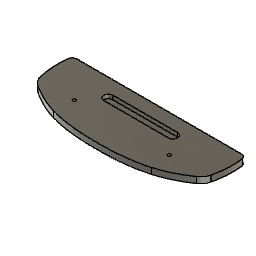
realsense_mounting (Autodesk Fusion 360 archive; units mm, degrees)
design "realsense_v2_partB_nowy"
Autodesk Fusion 360 part; units mm, degrees
sketch "Szkic1" plane through (0, 0, 48.2) normal (0, 0, -1) x (1, 0, 0)
  circle A0 centre (22, 4) radius 4.6
  circle A1 centre (-23, 4) radius 4.6
  circle A2 centre (-48, 23) radius 1.55
  circle A3 centre (47, 23) radius 1.55
  spline S0 degree 3 poles (86.9957, -10.4167) (86.9827, -10.5257) (86.9642, -10.6357) (86.8862, -10.9958) (86.803, -11.2409) (86.6033, -11.6873) (86.4654, -11.9278) (86.1402, -12.3732) (85.953, -12.5782) (85.5638, -12.9366) (85.323, -13.1197) (84.8088, -13.433) (84.5355, -13.5634) (83.9989, -13.7682) (83.6841, -13.8577) (83.043, -13.9736) (82.7166, -14) (82.4182, -14) knots 0.040108 0.040108 0.040108 0.040108 0.070809 0.070809 0.141618 0.141618 0.21753 0.21753 0.293443 0.293443 0.376236 0.376236 0.45903 0.45903 0.548548 0.548548 0.638067 0.638067 0.638067 0.638067
  arc A4 (86.9957, -10.4167) -> (85.4033, 19.5714) centre (0, 0) ccw
  spline S1 degree 3 poles (79.3689, 28.1539) (80.8996, 27.1108) (82.2391, 25.8176) (84.2935, 22.8681) (85.0138, 21.2712) (85.4033, 19.5714) knots 0 0 0 0 0.555691 0.555691 1.080379 1.080379 1.080379 1.080379
  spline S2 degree 3 poles (49.2048, 42.7622) (55.6443, 40.7737) (61.7849, 38.2476) (70.6441, 33.6178) (73.4694, 31.9794) (77.285, 29.5505) (78.3324, 28.8602) (79.3689, 28.1539) knots -3.94761 -3.94761 -3.94761 -3.94761 -1.930013 -1.930013 -0.949409 -0.949409 -0.573103 -0.573103 -0.573103 -0.573103
  spline S3 degree 3 poles (48.8426, 42.8691) (48.9015, 42.8525) (48.9603, 42.8355) (49.0811, 42.7999) (49.143, 42.7812) (49.2048, 42.7622) knots 0 0 0 0 0.018367 0.018367 0.03777 0.03777 0.03777 0.03777
  spline S4 degree 3 poles (-48.8426, 42.8691) (-40.6904, 45.1649) (-32.417, 46.5589) (-15.556, 48.2484) (-6.5081, 48.5581) (26.5202, 48.3443) (40.7394, 45.1512) (48.8426, 42.8691) knots -4.195538 -4.195538 -4.195538 -4.195538 -3.362301 -3.362301 -2.51673 -2.51673 -0.018698 -0.018698 -0.018698 -0.018698
  spline S5 degree 3 poles (-49.2048, 42.7622) (-49.143, 42.7812) (-49.0811, 42.7999) (-48.9603, 42.8355) (-48.9015, 42.8525) (-48.8426, 42.8691) knots 0 0 0 0 0.019402 0.019402 0.03777 0.03777 0.03777 0.03777
  spline S6 degree 3 poles (-79.3689, 28.1539) (-78.2934, 28.8868) (-77.2063, 29.6024) (-73.4168, 32.0083) (-70.6615, 33.6053) (-61.8482, 38.2216) (-55.6777, 40.7634) (-49.2048, 42.7622) knots -3.401993 -3.401993 -3.401993 -3.401993 -3.010569 -3.010569 -2.052057 -2.052057 -0.018974 -0.018974 -0.018974 -0.018974
  spline S7 degree 3 poles (-85.4033, 19.5714) (-85.0158, 21.2624) (-84.301, 22.8516) (-82.2522, 25.805) (-80.9072, 27.1057) (-79.3689, 28.1539) knots 0 0 0 0 0.520427 0.520427 1.077197 1.077197 1.077197 1.077197
  arc A5 (-85.4033, 19.5714) -> (-86.9957, -10.4167) centre (0, 0) ccw
  spline S8 degree 3 poles (-82.4182, -14) (-82.7166, -14) (-83.043, -13.9736) (-83.6841, -13.8577) (-83.9989, -13.7682) (-84.5355, -13.5634) (-84.8088, -13.433) (-85.323, -13.1197) (-85.5638, -12.9366) (-85.953, -12.5782) (-86.1402, -12.3732) (-86.4654, -11.9278) (-86.6033, -11.6873) (-86.803, -11.2409) (-86.8862, -10.9958) (-86.9642, -10.6357) (-86.9827, -10.5257) (-86.9957, -10.4167) knots 1.92305 1.92305 1.92305 1.92305 2.012569 2.012569 2.102087 2.102087 2.184881 2.184881 2.267674 2.267674 2.343587 2.343587 2.419499 2.419499 2.490308 2.490308 2.521009 2.521009 2.521009 2.521009
  line L0 (-82.4182, -14) -> (82.4182, -14)
extrude "Wyciągnięcie proste1" add sketch "Szkic1" along normal blind 5 makes body 1
sketch "Szkic2" plane through (0, 0, 48.2) normal (0, 0, 1) x (-1, 0, 0)
  circle A0 centre (-22, 4) radius 4.6
  circle A1 centre (48, 23) radius 1.55
  circle A2 centre (23, 4) radius 4.6
  circle A3 centre (-47, 23) radius 1.55
  arc A4 (86.9957, -10.4167) -> (85.4033, 19.5714) centre (0, 0) ccw
  spline S0 degree 3 poles (85.4033, 19.5714) (85.0158, 21.2624) (84.301, 22.8516) (82.2522, 25.805) (80.9072, 27.1057) (79.3689, 28.1539) knots 0 0 0 0 0.520427 0.520427 1.077197 1.077197 1.077197 1.077197
  spline S1 degree 3 poles (79.3689, 28.1539) (78.2934, 28.8868) (77.2063, 29.6024) (73.4168, 32.0083) (70.6615, 33.6053) (61.8482, 38.2216) (55.6777, 40.7634) (49.2048, 42.7622) knots -3.401993 -3.401993 -3.401993 -3.401993 -3.010569 -3.010569 -2.052057 -2.052057 -0.018974 -0.018974 -0.018974 -0.018974
  spline S2 degree 3 poles (49.2048, 42.7622) (49.143, 42.7812) (49.0811, 42.7999) (48.9603, 42.8355) (48.9015, 42.8525) (48.8426, 42.8691) knots 0 0 0 0 0.019402 0.019402 0.03777 0.03777 0.03777 0.03777
  spline S3 degree 3 poles (48.8426, 42.8691) (40.6904, 45.1649) (32.417, 46.5589) (15.556, 48.2484) (6.5081, 48.5581) (-26.5202, 48.3443) (-40.7394, 45.1512) (-48.8426, 42.8691) knots -4.195538 -4.195538 -4.195538 -4.195538 -3.362301 -3.362301 -2.51673 -2.51673 -0.018698 -0.018698 -0.018698 -0.018698
  spline S4 degree 3 poles (-48.8426, 42.8691) (-48.9015, 42.8525) (-48.9603, 42.8355) (-49.0811, 42.7999) (-49.143, 42.7812) (-49.2048, 42.7622) knots 0 0 0 0 0.018367 0.018367 0.03777 0.03777 0.03777 0.03777
  spline S5 degree 3 poles (-49.2048, 42.7622) (-55.6443, 40.7737) (-61.7849, 38.2476) (-70.6441, 33.6178) (-73.4694, 31.9794) (-77.285, 29.5505) (-78.3324, 28.8602) (-79.3689, 28.1539) knots -3.94761 -3.94761 -3.94761 -3.94761 -1.930013 -1.930013 -0.949409 -0.949409 -0.573103 -0.573103 -0.573103 -0.573103
  spline S6 degree 3 poles (-79.3689, 28.1539) (-80.8996, 27.1108) (-82.2391, 25.8176) (-84.2935, 22.8681) (-85.0138, 21.2712) (-85.4033, 19.5714) knots 0 0 0 0 0.555691 0.555691 1.080379 1.080379 1.080379 1.080379
  arc A5 (-85.4033, 19.5714) -> (-86.9957, -10.4167) centre (0, 0) ccw
  spline S7 degree 3 poles (-86.9957, -10.4167) (-86.9827, -10.5257) (-86.9642, -10.6357) (-86.8862, -10.9958) (-86.803, -11.2409) (-86.6033, -11.6873) (-86.4654, -11.9278) (-86.1402, -12.3732) (-85.953, -12.5782) (-85.5638, -12.9366) (-85.323, -13.1197) (-84.8088, -13.433) (-84.5355, -13.5634) (-83.9989, -13.7682) (-83.6841, -13.8577) (-83.043, -13.9736) (-82.7166, -14) (-82.4182, -14) knots 0.040108 0.040108 0.040108 0.040108 0.070809 0.070809 0.141618 0.141618 0.21753 0.21753 0.293443 0.293443 0.376236 0.376236 0.45903 0.45903 0.548548 0.548548 0.638067 0.638067 0.638067 0.638067
  line L0 (-82.4182, -14) -> (82.4182, -14)
  spline S8 degree 3 poles (82.4182, -14) (82.7166, -14) (83.043, -13.9736) (83.6841, -13.8577) (83.9989, -13.7682) (84.5355, -13.5634) (84.8088, -13.433) (85.323, -13.1197) (85.5638, -12.9366) (85.953, -12.5782) (86.1402, -12.3732) (86.4654, -11.9278) (86.6033, -11.6873) (86.803, -11.2409) (86.8862, -10.9958) (86.9642, -10.6357) (86.9827, -10.5257) (86.9957, -10.4167) knots 1.92305 1.92305 1.92305 1.92305 2.012569 2.012569 2.102087 2.102087 2.184881 2.184881 2.267674 2.267674 2.343587 2.343587 2.419499 2.419499 2.490308 2.490308 2.521009 2.521009 2.521009 2.521009
  line L1 (-22, 4) -> (23, 4)
  line L2 (23, 4) -> (23, 8.6)
  line L3 (23, 8.6) -> (-22, 8.6)
  line L4 (-22, 8.6) -> (-22, 4)
  line L5 (23, 4) -> (-22, 4)
  line L6 (-22, 4) -> (-22, -0.6)
  line L7 (-22, -0.6) -> (23, -0.6)
  line L8 (23, -0.6) -> (23, 4)
  line L9 (-22, 4) -> (-32, 4)
  line L10 (23, 4) -> (33, 4)
  line L11 (-22, -0.6) -> (-32, -0.6)
  line L12 (-32, -0.6) -> (-32, 4)
  line L13 (-32, 4) -> (-22, 4)
  line L14 (-22, 4) -> (-22, -0.6)
  line L15 (-22, 8.6) -> (-32, 8.6)
  line L16 (-32, 8.6) -> (-32, 4)
  line L17 (-32, 4) -> (-22, 4)
  line L18 (-22, 4) -> (-22, 8.6)
  line L19 (23, 8.6) -> (33, 8.6)
  line L20 (33, 8.6) -> (33, 4)
  line L21 (33, 4) -> (23, 4)
  line L22 (23, 4) -> (23, 8.6)
  line L23 (23, -0.6) -> (33, -0.6)
  line L24 (33, -0.6) -> (33, 4)
  line L25 (33, 4) -> (23, 4)
  line L26 (23, 4) -> (23, -0.6)
  circle A6 centre (-32, 4) radius 4.6
  circle A7 centre (33, 4) radius 4.6
  dimension "d3" = 10
  dimension "d4" = 10
  constraint horizontal L1
  constraint vertical L2
  constraint horizontal L3
  constraint vertical L4
  constraint coincident A2 L2.end
  constraint coincident A0.centre L1.start
  constraint horizontal L5
  constraint vertical L6
  constraint horizontal L7
  constraint vertical L8
  constraint coincident A0 L6.end
  constraint perpendicular L6 L9
  constraint perpendicular L8 L10
  constraint horizontal L11
  constraint vertical L12
  constraint horizontal L13
  constraint vertical L14
  constraint horizontal L15
  constraint vertical L16
  constraint horizontal L17
  constraint vertical L18
  constraint horizontal L19
  constraint vertical L20
  constraint horizontal L21
  constraint vertical L22
  constraint horizontal L23
  constraint vertical L24
  constraint horizontal L25
  constraint vertical L26
  constraint coincident L9.end L12.end
  constraint coincident L15.end A6
  constraint coincident L10.end L20.end
  constraint coincident L19.end A7
  measures "d3" distance of A0.centre L9.end
  measures "d4" distance of A2.centre L10.end
extrude "Wyciągnięcie proste2" add sketch "Szkic2" against normal blind 4 separate body contours A0 L1 L4 L5 L18 | A0 A2 L1 L5 L7 | A0 L1 L5 L6 L14 | A0 A2 L1 L3 L5 | A0 L4 L9 L13 L17 L18 | A0 L9 L13 L15 L17 A6 | A0 L9 L11 L13 L17 A6 | A0 L6 L9 L13 L14 L17 | A2 L1 L5 L8 L26 | A2 L1 L2 L5 L22 | A2 L10 L19 L21 L25 A7 | A2 L2 L10 L21 L22 L25 | L9 L13 L16 L17 A6 | L12 L16 A6 | A2 L8 L10 L21 L25 L26 | A2 L10 L21 L23 L25 A7 | L9 L12 L13 L17 A6 | L20 L24 A7 | L10 L20 L21 L25 A7 | L10 L21 L24 L25 A7 makes body 2
delete_face "Usuń powierzchnię1" 1 faces at (26.5771, -3.542, 46.5333) on bodies 1
delete_face "Usuń powierzchnię2" 1 faces at (-18.4229, -3.542, 46.5333) on bodies 1
sketch "Szkic3" plane through (0, 0, 48.2) normal (0, 0, 1) x (-1, 0, 0)
  circle A0 centre (48, 23) radius 1.55
  circle A1 centre (-47, 23) radius 1.55
  arc A2 (86.9957, -10.4167) -> (85.4033, 19.5714) centre (0, 0) ccw
  spline S0 degree 3 poles (85.4033, 19.5714) (85.0158, 21.2624) (84.301, 22.8516) (82.2522, 25.805) (80.9072, 27.1057) (79.3689, 28.1539) knots 0 0 0 0 0.520427 0.520427 1.077197 1.077197 1.077197 1.077197
  spline S1 degree 3 poles (79.3689, 28.1539) (78.2934, 28.8868) (77.2063, 29.6024) (73.4168, 32.0083) (70.6615, 33.6053) (61.8482, 38.2216) (55.6777, 40.7634) (49.2048, 42.7622) knots -3.401993 -3.401993 -3.401993 -3.401993 -3.010569 -3.010569 -2.052057 -2.052057 -0.018974 -0.018974 -0.018974 -0.018974
  spline S2 degree 3 poles (49.2048, 42.7622) (49.143, 42.7812) (49.0811, 42.7999) (48.9603, 42.8355) (48.9015, 42.8525) (48.8426, 42.8691) knots 0 0 0 0 0.019402 0.019402 0.03777 0.03777 0.03777 0.03777
  spline S3 degree 3 poles (48.8426, 42.8691) (40.6904, 45.1649) (32.417, 46.5589) (15.556, 48.2484) (6.5081, 48.5581) (-26.5202, 48.3443) (-40.7394, 45.1512) (-48.8426, 42.8691) knots -4.195538 -4.195538 -4.195538 -4.195538 -3.362301 -3.362301 -2.51673 -2.51673 -0.018698 -0.018698 -0.018698 -0.018698
  spline S4 degree 3 poles (-48.8426, 42.8691) (-48.9015, 42.8525) (-48.9603, 42.8355) (-49.0811, 42.7999) (-49.143, 42.7812) (-49.2048, 42.7622) knots 0 0 0 0 0.018367 0.018367 0.03777 0.03777 0.03777 0.03777
  spline S5 degree 3 poles (-49.2048, 42.7622) (-55.6443, 40.7737) (-61.7849, 38.2476) (-70.6441, 33.6178) (-73.4694, 31.9794) (-77.285, 29.5505) (-78.3324, 28.8602) (-79.3689, 28.1539) knots -3.94761 -3.94761 -3.94761 -3.94761 -1.930013 -1.930013 -0.949409 -0.949409 -0.573103 -0.573103 -0.573103 -0.573103
  spline S6 degree 3 poles (-79.3689, 28.1539) (-80.8996, 27.1108) (-82.2391, 25.8176) (-84.2935, 22.8681) (-85.0138, 21.2712) (-85.4033, 19.5714) knots 0 0 0 0 0.555691 0.555691 1.080379 1.080379 1.080379 1.080379
  arc A3 (-85.4033, 19.5714) -> (-86.9957, -10.4167) centre (0, 0) ccw
  spline S7 degree 3 poles (-86.9957, -10.4167) (-86.9827, -10.5257) (-86.9642, -10.6357) (-86.8862, -10.9958) (-86.803, -11.2409) (-86.6033, -11.6873) (-86.4654, -11.9278) (-86.1402, -12.3732) (-85.953, -12.5782) (-85.5638, -12.9366) (-85.323, -13.1197) (-84.8088, -13.433) (-84.5355, -13.5634) (-83.9989, -13.7682) (-83.6841, -13.8577) (-83.043, -13.9736) (-82.7166, -14) (-82.4182, -14) knots 0.040108 0.040108 0.040108 0.040108 0.070809 0.070809 0.141618 0.141618 0.21753 0.21753 0.293443 0.293443 0.376236 0.376236 0.45903 0.45903 0.548548 0.548548 0.638067 0.638067 0.638067 0.638067
  line L0 (-82.4182, -14) -> (82.4182, -14)
  spline S8 degree 3 poles (82.4182, -14) (82.7166, -14) (83.043, -13.9736) (83.6841, -13.8577) (83.9989, -13.7682) (84.5355, -13.5634) (84.8088, -13.433) (85.323, -13.1197) (85.5638, -12.9366) (85.953, -12.5782) (86.1402, -12.3732) (86.4654, -11.9278) (86.6033, -11.6873) (86.803, -11.2409) (86.8862, -10.9958) (86.9642, -10.6357) (86.9827, -10.5257) (86.9957, -10.4167) knots 1.92305 1.92305 1.92305 1.92305 2.012569 2.012569 2.102087 2.102087 2.184881 2.184881 2.267674 2.267674 2.343587 2.343587 2.419499 2.419499 2.490308 2.490308 2.521009 2.521009 2.521009 2.521009
  line L1 (-43.945, 23) -> (-45.4725, 25.6457)
  line L2 (-45.4725, 25.6457) -> (-48.5275, 25.6457)
  line L3 (-48.5275, 25.6457) -> (-50.055, 23)
  line L4 (-50.055, 23) -> (-48.5275, 20.3543)
  line L5 (-48.5275, 20.3543) -> (-45.4725, 20.3543)
  line L6 (-45.4725, 20.3543) -> (-43.945, 23)
  line L7 (51.055, 23) -> (49.5275, 25.6457)
  line L8 (49.5275, 25.6457) -> (46.4725, 25.6457)
  line L9 (46.4725, 25.6457) -> (44.945, 23)
  line L10 (44.945, 23) -> (46.4725, 20.3543)
  line L11 (46.4725, 20.3543) -> (49.5275, 20.3543)
  line L12 (49.5275, 20.3543) -> (51.055, 23)
  point P0 (-47, 23)
  point P1 (-47, 23)
  point P2 (48, 23)
  dimension "d7" = 3.055
  dimension "d8" = 3.055
  constraint coincident P1 P0
  constraint coincident P2 A0.centre
  measures "d7" distance of L1.start P1
  measures "d8" distance of L7.start P2
extrude "Wyciągnięcie proste3" add sketch "Szkic3" against normal blind 2.5 separate body contours L1 L2 L3 L4 L5 L6 | L7 L8 L9 L10 L11 L12 makes body 3 at (47.0386, -24.5495, 46.5333) makes body 4 at (-47.9614, -24.5495, 46.5333)
extrude "Wyciągnięcie proste4" add 1 faces at (15.4083, 2.1141, 43.2) along direction (0, 0, -1) blind 1 on bodies 1 bodies 1
move_body "Przesuń2" bodies 3 4 to x (1, 0, 0) y (0, 1, 0) z (0, 0, 1) at (0, 0, -2.5)
combine "Kombinacja2" operation cut target body 1 tool bodies 2 3 4
sketch "Szkic4" plane through (0, 0, 42.2) normal (0, 0, -1) x (1, 0, 0)
  circle A0 centre (-48, 23) radius 1.55
  circle A1 centre (47, 23) radius 1.55
  arc A2 (-85.4033, 19.5714) -> (-86.9957, -10.4167) centre (0, 0) ccw
  spline S0 degree 3 poles (-86.9957, -10.4167) (-86.9827, -10.5257) (-86.9642, -10.6357) (-86.8862, -10.9958) (-86.803, -11.2409) (-86.6033, -11.6873) (-86.4654, -11.9278) (-86.1402, -12.3732) (-85.953, -12.5782) (-85.5638, -12.9366) (-85.323, -13.1197) (-84.8088, -13.433) (-84.5355, -13.5634) (-83.9989, -13.7682) (-83.6841, -13.8577) (-83.043, -13.9736) (-82.7166, -14) (-82.4182, -14) knots -2.521009 -2.521009 -2.521009 -2.521009 -2.490308 -2.490308 -2.419499 -2.419499 -2.343587 -2.343587 -2.267674 -2.267674 -2.184881 -2.184881 -2.102087 -2.102087 -2.012569 -2.012569 -1.92305 -1.92305 -1.92305 -1.92305
  line L0 (-82.4182, -14) -> (82.4182, -14)
  spline S1 degree 3 poles (82.4182, -14) (82.7166, -14) (83.043, -13.9736) (83.6841, -13.8577) (83.9989, -13.7682) (84.5355, -13.5634) (84.8088, -13.433) (85.323, -13.1197) (85.5638, -12.9366) (85.953, -12.5782) (86.1402, -12.3732) (86.4654, -11.9278) (86.6033, -11.6873) (86.803, -11.2409) (86.8862, -10.9958) (86.9642, -10.6357) (86.9827, -10.5257) (86.9957, -10.4167) knots -0.638067 -0.638067 -0.638067 -0.638067 -0.548548 -0.548548 -0.45903 -0.45903 -0.376236 -0.376236 -0.293443 -0.293443 -0.21753 -0.21753 -0.141618 -0.141618 -0.070809 -0.070809 -0.040108 -0.040108 -0.040108 -0.040108
  arc A3 (86.9957, -10.4167) -> (85.4033, 19.5714) centre (0, 0) ccw
  spline S2 degree 3 poles (85.4033, 19.5714) (85.0138, 21.2712) (84.2935, 22.8681) (82.2391, 25.8176) (80.8996, 27.1108) (79.3689, 28.1539) knots -1.080379 -1.080379 -1.080379 -1.080379 -0.555691 -0.555691 0 0 0 0
  spline S3 degree 3 poles (79.3689, 28.1539) (78.3324, 28.8602) (77.285, 29.5505) (73.4694, 31.9794) (70.6441, 33.6178) (61.7849, 38.2476) (55.6443, 40.7737) (49.2048, 42.7622) knots 0.573103 0.573103 0.573103 0.573103 0.949409 0.949409 1.930013 1.930013 3.94761 3.94761 3.94761 3.94761
  spline S4 degree 3 poles (49.2048, 42.7622) (49.143, 42.7812) (49.0811, 42.7999) (48.9603, 42.8355) (48.9015, 42.8525) (48.8426, 42.8691) knots -0.03777 -0.03777 -0.03777 -0.03777 -0.018367 -0.018367 0 0 0 0
  spline S5 degree 3 poles (48.8426, 42.8691) (40.7394, 45.1512) (26.5202, 48.3443) (-6.5081, 48.5581) (-15.556, 48.2484) (-32.417, 46.5589) (-40.6904, 45.1649) (-48.8426, 42.8691) knots 0.018698 0.018698 0.018698 0.018698 2.51673 2.51673 3.362301 3.362301 4.195538 4.195538 4.195538 4.195538
  spline S6 degree 3 poles (-48.8426, 42.8691) (-48.9015, 42.8525) (-48.9603, 42.8355) (-49.0811, 42.7999) (-49.143, 42.7812) (-49.2048, 42.7622) knots -0.03777 -0.03777 -0.03777 -0.03777 -0.019402 -0.019402 0 0 0 0
  spline S7 degree 3 poles (-49.2048, 42.7622) (-55.6777, 40.7634) (-61.8482, 38.2216) (-70.6615, 33.6053) (-73.4168, 32.0083) (-77.2063, 29.6024) (-78.2934, 28.8868) (-79.3689, 28.1539) knots 0.018974 0.018974 0.018974 0.018974 2.052057 2.052057 3.010569 3.010569 3.401993 3.401993 3.401993 3.401993
  spline S8 degree 3 poles (-79.3689, 28.1539) (-80.9072, 27.1057) (-82.2522, 25.805) (-84.301, 22.8516) (-85.0158, 21.2624) (-85.4033, 19.5714) knots -1.077197 -1.077197 -1.077197 -1.077197 -0.520427 -0.520427 0 0 0 0
  line L1 (-50, 25) -> (50, 25)
  line L2 (50, 25) -> (50, 20)
  line L3 (50, 20) -> (-50, 20)
  line L4 (-50, 20) -> (-50, 25)
  constraint horizontal L1
  constraint vertical L2
  constraint horizontal L3
  constraint vertical L4
sketch "Szkic5" plane through (0, 0, 42.2) normal (0, 0, -1) x (1, 0, 0)
  circle A0 centre (-48, 23) radius 1.55
  circle A1 centre (47, 23) radius 1.55
  arc A2 (-85.4033, 19.5714) -> (-86.9957, -10.4167) centre (0, 0) ccw
  spline S0 degree 3 poles (-86.9957, -10.4167) (-86.9827, -10.5257) (-86.9642, -10.6357) (-86.8862, -10.9958) (-86.803, -11.2409) (-86.6033, -11.6873) (-86.4654, -11.9278) (-86.1402, -12.3732) (-85.953, -12.5782) (-85.5638, -12.9366) (-85.323, -13.1197) (-84.8088, -13.433) (-84.5355, -13.5634) (-83.9989, -13.7682) (-83.6841, -13.8577) (-83.043, -13.9736) (-82.7166, -14) (-82.4182, -14) knots -2.521009 -2.521009 -2.521009 -2.521009 -2.490308 -2.490308 -2.419499 -2.419499 -2.343587 -2.343587 -2.267674 -2.267674 -2.184881 -2.184881 -2.102087 -2.102087 -2.012569 -2.012569 -1.92305 -1.92305 -1.92305 -1.92305
  line L0 (-82.4182, -14) -> (82.4182, -14)
  spline S1 degree 3 poles (82.4182, -14) (82.7166, -14) (83.043, -13.9736) (83.6841, -13.8577) (83.9989, -13.7682) (84.5355, -13.5634) (84.8088, -13.433) (85.323, -13.1197) (85.5638, -12.9366) (85.953, -12.5782) (86.1402, -12.3732) (86.4654, -11.9278) (86.6033, -11.6873) (86.803, -11.2409) (86.8862, -10.9958) (86.9642, -10.6357) (86.9827, -10.5257) (86.9957, -10.4167) knots -0.638067 -0.638067 -0.638067 -0.638067 -0.548548 -0.548548 -0.45903 -0.45903 -0.376236 -0.376236 -0.293443 -0.293443 -0.21753 -0.21753 -0.141618 -0.141618 -0.070809 -0.070809 -0.040108 -0.040108 -0.040108 -0.040108
  arc A3 (86.9957, -10.4167) -> (85.4033, 19.5714) centre (0, 0) ccw
  spline S2 degree 3 poles (85.4033, 19.5714) (85.0138, 21.2712) (84.2935, 22.8681) (82.2391, 25.8176) (80.8996, 27.1108) (79.3689, 28.1539) knots -1.080379 -1.080379 -1.080379 -1.080379 -0.555691 -0.555691 0 0 0 0
  spline S3 degree 3 poles (79.3689, 28.1539) (78.3324, 28.8602) (77.285, 29.5505) (73.4694, 31.9794) (70.6441, 33.6178) (61.7849, 38.2476) (55.6443, 40.7737) (49.2048, 42.7622) knots 0.573103 0.573103 0.573103 0.573103 0.949409 0.949409 1.930013 1.930013 3.94761 3.94761 3.94761 3.94761
  spline S4 degree 3 poles (49.2048, 42.7622) (49.143, 42.7812) (49.0811, 42.7999) (48.9603, 42.8355) (48.9015, 42.8525) (48.8426, 42.8691) knots -0.03777 -0.03777 -0.03777 -0.03777 -0.018367 -0.018367 0 0 0 0
  spline S5 degree 3 poles (48.8426, 42.8691) (40.7394, 45.1512) (26.5202, 48.3443) (-6.5081, 48.5581) (-15.556, 48.2484) (-32.417, 46.5589) (-40.6904, 45.1649) (-48.8426, 42.8691) knots 0.018698 0.018698 0.018698 0.018698 2.51673 2.51673 3.362301 3.362301 4.195538 4.195538 4.195538 4.195538
  spline S6 degree 3 poles (-48.8426, 42.8691) (-48.9015, 42.8525) (-48.9603, 42.8355) (-49.0811, 42.7999) (-49.143, 42.7812) (-49.2048, 42.7622) knots -0.03777 -0.03777 -0.03777 -0.03777 -0.019402 -0.019402 0 0 0 0
  spline S7 degree 3 poles (-49.2048, 42.7622) (-55.6777, 40.7634) (-61.8482, 38.2216) (-70.6615, 33.6053) (-73.4168, 32.0083) (-77.2063, 29.6024) (-78.2934, 28.8868) (-79.3689, 28.1539) knots 0.018974 0.018974 0.018974 0.018974 2.052057 2.052057 3.010569 3.010569 3.401993 3.401993 3.401993 3.401993
  spline S8 degree 3 poles (-79.3689, 28.1539) (-80.9072, 27.1057) (-82.2522, 25.805) (-84.301, 22.8516) (-85.0158, 21.2624) (-85.4033, 19.5714) knots -1.077197 -1.077197 -1.077197 -1.077197 -0.520427 -0.520427 0 0 0 0
extrude "Wyciągnięcie proste5" add sketch "Szkic4" against normal blind 1 separate body contours L1 L2 L3 L4 makes body 5
delete_face "Usuń powierzchnię3" 1 faces at (-47.9614, -24.5495, 42.8667) on bodies 5
delete_face "Usuń powierzchnię4" 1 faces at (47.0386, -24.5495, 42.8667) on bodies 5
combine "Kombinacja3" operation add target body 1 tool bodies 5
extrude "Wyciągnięcie proste6" add 4 faces at (-47.9614, -20.721, 43.2) (-50.3517, -23, 43.2) (-47.4908, -25.2152, 43.2) (-48.115, -23.5037, 43.2) along direction (0, 0, 1) blind 0.1 on bodies 1 bodies 1
extrude "Wyciągnięcie proste7" add 4 faces at (45.007, -21.8939, 43.2) (50.0183, -23, 43.2) (46.4908, -25.2152, 43.2) (46.885, -23.5037, 43.2) along direction (0, 0, 1) blind 0.1 on bodies 1 bodies 1
sketch "Szkic6" plane through (0, 0, 43.3) normal (0, 0, 1) x (-1, 0, 0)
  line L0 (-48.5275, 25.6457) -> (-50.055, 23)
  line L1 (-50.055, 23) -> (-48.5275, 20.3543)
  line L2 (-48.5275, 20.3543) -> (-45.4725, 20.3543)
  line L3 (-45.4725, 20.3543) -> (-43.945, 23)
  line L4 (-43.945, 23) -> (-45.4725, 25.6457)
  line L5 (-45.4725, 25.6457) -> (-48.5275, 25.6457)
  point P0 (-47, 23)
  point P1 (-47, 23)
sketch "Szkic7" plane through (0, 0, 48.2) normal (0, 0, 1) x (-1, 0, 0)
  arc A0 (33, -0.6) -> (33, 8.6) centre (33, 4) ccw
  line L0 (33, -0.6) -> (-32, -0.6)
  arc A1 (-32, 8.6) -> (-32, -0.6) centre (-32, 4) ccw
  line L1 (-32, 8.6) -> (33, 8.6)
  circle A2 centre (48, 23) radius 1.55
  circle A3 centre (-47, 23) radius 1.55
  arc A4 (86.9957, -10.4167) -> (85.4033, 19.5714) centre (0, 0) ccw
  spline S0 degree 3 poles (85.4033, 19.5714) (85.0158, 21.2624) (84.301, 22.8516) (82.2522, 25.805) (80.9072, 27.1057) (79.3689, 28.1539) knots 0 0 0 0 0.520427 0.520427 1.077197 1.077197 1.077197 1.077197
  spline S1 degree 3 poles (79.3689, 28.1539) (78.2934, 28.8868) (77.2063, 29.6024) (73.4168, 32.0083) (70.6615, 33.6053) (61.8482, 38.2216) (55.6777, 40.7634) (49.2048, 42.7622) knots -3.401993 -3.401993 -3.401993 -3.401993 -3.010569 -3.010569 -2.052057 -2.052057 -0.018974 -0.018974 -0.018974 -0.018974
  spline S2 degree 3 poles (49.2048, 42.7622) (49.143, 42.7812) (49.0811, 42.7999) (48.9603, 42.8355) (48.9015, 42.8525) (48.8426, 42.8691) knots 0 0 0 0 0.019402 0.019402 0.03777 0.03777 0.03777 0.03777
  spline S3 degree 3 poles (48.8426, 42.8691) (40.6904, 45.1649) (32.417, 46.5589) (15.556, 48.2484) (6.5081, 48.5581) (-26.5202, 48.3443) (-40.7394, 45.1512) (-48.8426, 42.8691) knots -4.195538 -4.195538 -4.195538 -4.195538 -3.362301 -3.362301 -2.51673 -2.51673 -0.018698 -0.018698 -0.018698 -0.018698
  spline S4 degree 3 poles (-48.8426, 42.8691) (-48.9015, 42.8525) (-48.9603, 42.8355) (-49.0811, 42.7999) (-49.143, 42.7812) (-49.2048, 42.7622) knots 0 0 0 0 0.018367 0.018367 0.03777 0.03777 0.03777 0.03777
  spline S5 degree 3 poles (-49.2048, 42.7622) (-55.6443, 40.7737) (-61.7849, 38.2476) (-70.6441, 33.6178) (-73.4694, 31.9794) (-77.285, 29.5505) (-78.3324, 28.8602) (-79.3689, 28.1539) knots -3.94761 -3.94761 -3.94761 -3.94761 -1.930013 -1.930013 -0.949409 -0.949409 -0.573103 -0.573103 -0.573103 -0.573103
  spline S6 degree 3 poles (-79.3689, 28.1539) (-80.8996, 27.1108) (-82.2391, 25.8176) (-84.2935, 22.8681) (-85.0138, 21.2712) (-85.4033, 19.5714) knots 0 0 0 0 0.555691 0.555691 1.080379 1.080379 1.080379 1.080379
  arc A5 (-85.4033, 19.5714) -> (-86.9957, -10.4167) centre (0, 0) ccw
  spline S7 degree 3 poles (-86.9957, -10.4167) (-86.9827, -10.5257) (-86.9642, -10.6357) (-86.8862, -10.9958) (-86.803, -11.2409) (-86.6033, -11.6873) (-86.4654, -11.9278) (-86.1402, -12.3732) (-85.953, -12.5782) (-85.5638, -12.9366) (-85.323, -13.1197) (-84.8088, -13.433) (-84.5355, -13.5634) (-83.9989, -13.7682) (-83.6841, -13.8577) (-83.043, -13.9736) (-82.7166, -14) (-82.4182, -14) knots 0.040108 0.040108 0.040108 0.040108 0.070809 0.070809 0.141618 0.141618 0.21753 0.21753 0.293443 0.293443 0.376236 0.376236 0.45903 0.45903 0.548548 0.548548 0.638067 0.638067 0.638067 0.638067
  line L2 (-82.4182, -14) -> (82.4182, -14)
  spline S8 degree 3 poles (82.4182, -14) (82.7166, -14) (83.043, -13.9736) (83.6841, -13.8577) (83.9989, -13.7682) (84.5355, -13.5634) (84.8088, -13.433) (85.323, -13.1197) (85.5638, -12.9366) (85.953, -12.5782) (86.1402, -12.3732) (86.4654, -11.9278) (86.6033, -11.6873) (86.803, -11.2409) (86.8862, -10.9958) (86.9642, -10.6357) (86.9827, -10.5257) (86.9957, -10.4167) knots 1.92305 1.92305 1.92305 1.92305 2.012569 2.012569 2.102087 2.102087 2.184881 2.184881 2.267674 2.267674 2.343587 2.343587 2.419499 2.419499 2.490308 2.490308 2.521009 2.521009 2.521009 2.521009
  circle A6 centre (-47, 23) radius 1.55
  circle A7 centre (48, 23) radius 1.55
  constraint concentric A3 A6
  constraint concentric A2 A7
extrude "Wyciągnięcie proste8" add sketch "Szkic7" against normal blind 5.4 separate body contours A2 A7 | A3 A6 makes body 6 at (-47.9614, -24.5495, 44.6) makes body 7 at (47.0386, -24.5495, 44.6)
combine "Kombinacja4" operation cut target body 1 tool bodies 6 7
extrude "Wyciągnięcie proste9" cut 2 faces at (45.0456, -21.827, 43.3) (-46.007, -21.8939, 43.3) along direction (0, 0, -1) blind 0.2 on bodies 1 bodies 1
sketch "Szkic10" plane through (0, 0, 43.1) normal (0, 0, 1) x (-1, 0, 0)
  circle A0 centre (48, 23) radius 1.55
  line L0 (51.055, 23) -> (49.5275, 25.6457)
  line L1 (49.5275, 25.6457) -> (46.4725, 25.6457)
  line L2 (46.4725, 25.6457) -> (44.945, 23)
  line L3 (44.945, 23) -> (46.4725, 20.3543)
  line L4 (46.4725, 20.3543) -> (49.5275, 20.3543)
  line L5 (49.5275, 20.3543) -> (51.055, 23)
  line L6 (44.65, 23) -> (46.325, 20.0988)
  line L7 (46.325, 20.0988) -> (49.675, 20.0988)
  line L8 (49.675, 20.0988) -> (51.35, 23)
  line L9 (51.35, 23) -> (49.675, 25.9012)
  line L10 (49.675, 25.9012) -> (46.325, 25.9012)
  line L11 (46.325, 25.9012) -> (44.65, 23)
  line L12 (-43.65, 23) -> (-45.325, 25.9012)
  line L13 (-45.325, 25.9012) -> (-48.675, 25.9012)
  line L14 (-48.675, 25.9012) -> (-50.35, 23)
  line L15 (-50.35, 23) -> (-48.675, 20.0988)
  line L16 (-48.675, 20.0988) -> (-45.325, 20.0988)
  line L17 (-45.325, 20.0988) -> (-43.65, 23)
  point P0 (48, 23)
  point P1 (-47, 23)
  dimension "d26" = 3.35
  dimension "d27" = 3.35
  constraint coincident P0 A0.centre
  measures "d26" distance of L6.start P0
  measures "d27" distance of L12.start P1
extrude "Wyciągnięcie proste10" add sketch "Szkic10" along normal blind 2.6 separate body contours A0 | L0 L1 L2 L3 L4 L5 | L6 L7 L8 L9 L10 L11 | L12 L13 L14 L15 L16 L17 makes body 8 at (-47.4417, -23.9671, 43.1) makes body 9 at (46.4417, -22.0329, 43.1)
combine "Kombinacja5" operation cut target body 1 tool bodies 8 9
